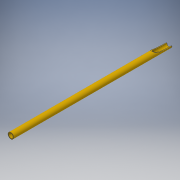
# Autodesk Inventor part: pin
Saved by Autodesk Inventor 2018 (Build 220112000, 112)
## iProperties
Created: 2019-04-17
Part Number: pin
Material: Generic
Document SubType Name: Modeling
Designer: ZEUSLAP
Density: 1 g/cm^3
Appearance: Default
Author: ZEUSLAP
Autodesk Inventor part; units mm, degrees
ref_plane "YZ Plane" through (0, 0, 0) normal (1, 0, 0) x (0, 1, 0)
ref_plane "XZ Plane" through (0, 0, 0) normal (0, 1, 0) x (-1, 0, 0)
ref_plane "XY Plane" through (0, 0, 0) normal (0, 0, 1) x (1, 0, 0)
sketch "Sketch1" plane through (0, 0, 0) normal (0, 1, 0) x (-1, 0, 0)
  circle A0 centre (0, 0) radius 0.5
  circle A1 centre (0, 0) radius 0.375
  dimension "d0" = 1
  dimension "d1" = 0.75
  constraints: 2 centre point, 2 coincident
  measures "d0" diameter of A0
  measures "d1" diameter of A1
extrude "Extrusion1" add sketch "Sketch1" along normal blind 27
sketch "Sketch2" plane through (0, 0, 0) normal (1, 0, 0) x (0, 1, 0)
  line L0 (0, 0.5) -> (27, 0.5) construction
  line L1 (27, -0.5) -> (24.5005, -0.5) construction
  line L2 (24, 0.5) -> (27.2057, 2.2706)
  line L3 (24, 0.5) -> (24.5005, 0) construction
  line L4 (24.5005, 0) -> (27, 0) construction
  spline S0 degree 2 poles (24, 0.5) (24.5005, 0) (27, 0) knots 1 1 1 2 2 2
  line L5 (27.2057, 2.2706) -> (27.2355, -0.0268)
  line L6 (27.2355, -0.0268) -> (27, 0)
  point P0 (0, 0)
  constraints: 8 end point, 1 horizontal, 1 parallel, 1 point on line, 3 other
extrude "Extrusion2" cut sketch "Sketch2" against normal blind 1 and the other way blind 1
body "Solid1"
